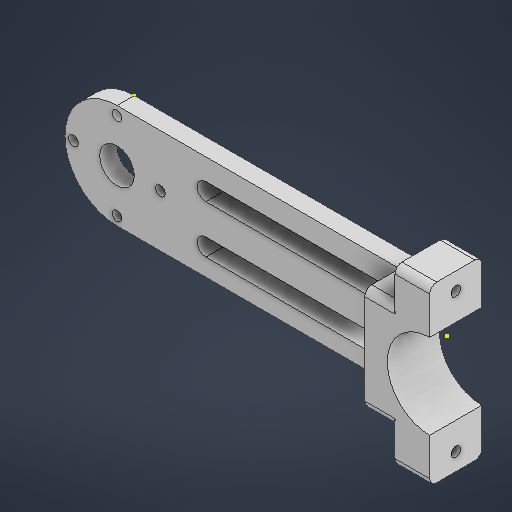
# Autodesk Inventor part: link1
Saved by Autodesk Inventor 2026.1 (Build 301233020, 233B)
## iProperties
Created: 2026-04-16
Part Number: link1
Material: Generic
Document SubType Name: Modeling
Designer: kadir
Density: 1 g/cm^3
Appearance: Default
Author: kadir
Autodesk Inventor part; units mm, degrees
ref_plane "YZ Plane" through (0, 0, 0) normal (1, 0, 0) x (0, 1, 0)
ref_plane "XZ Plane" through (0, 0, 0) normal (0, 1, 0) x (-1, 0, 0)
ref_plane "XY Plane" through (0, 0, 0) normal (0, 0, 1) x (1, 0, 0)
sketch "Sketch1" plane through (0, 0, 0) normal (0, 0, 1) x (1, 0, 0)
  circle A0 centre (0, 0) radius 15
  circle A1 centre (0, 0) radius 5
  circle A2 centre (-12.5, 0) radius 1.4
  circle A3 centre (0, -12.5) radius 1.4
  circle A4 centre (12.5, 0) radius 1.4
  circle A5 centre (0, 12.5) radius 1.4
  line L0 (0, -15) -> (1.0439, -14.9636)
  line L1 (100, 15) -> (70, 15)
  line L2 (70, -12.5614) -> (70, -15)
  line L3 (70, -15) -> (100, -15)
  line L4 (100, -15) -> (100, 15)
  line L5 (100, 15) -> (70, -15) construction
  line L6 (70, 15) -> (100, -15) construction
  circle A6 centre (100, 0) radius 12.2
  line L7 (0, 15) -> (100, 15)
  line L8 (0, -15) -> (100, -15)
  point P0 (85, 0)
  point P1 (100, -12.2)
  point P2 (100, 12.2)
  dimension "d0" = 30
  dimension "d1" = 10
  dimension "d2" = 2.8
  dimension "d3" = 12.5
  dimension "d6" = 360
  dimension "d9" = 30
  dimension "d10" = 30
  dimension "d11" = 24.4
  dimension "d12" = 100
  constraints: 18 end point, 7 centre point, 3 midpoint, 3 point on circle, 2 coincident, 2 horizontal alignment, 2 parallel, 1 horizontal, 1 perpendicular, 1 point on line, 1 tangent, 9 other
  measures "d0" diameter of A0
  measures "d1" diameter of A1
  measures "d2" diameter of A2
  measures "d3" distance of point (0, 0) A2.centre
  measures "d9" distance of L3.end L2.end
  measures "d10" distance of L2.end L1.end
  measures "d11" diameter of A6
  measures "d12" distance of A6.centre point (0, 0)
extrude "Extrusion1" add sketch "Sketch1" along normal blind 5 contours A0 L0 | A0 L7 L1 L4 A6 L3 L8 picked at (9.3778, -4.158)
sketch "Sketch2" plane through (0, 15, 0) normal (0, 1, 0) x (1, 0, 0)
  point P0 (0, 0)
sketch "Sketch3" plane through (0, 0, 5) normal (0, 0, 1) x (1, 0, 0)
  line L0 (100, 15) -> (0, 15) projected
  line L1 (0, -15) -> (100, -15) projected
  line L2 (81.3075, 15) -> (100, 15)
  line L3 (100, 15) -> (100, -15)
  line L4 (100, -15) -> (81.3075, -15)
  line L5 (81.3075, -15) -> (81.3075, 15)
  circle A0 centre (100, 0) radius 12.2
  point P0 (0, 0)
  point P1 (100, -12.2)
  point P2 (100, 12.2)
  dimension "d15" = 24.4
  constraints: 8 end point, 2 parallel, 1 centre point, 1 horizontal, 1 midpoint, 1 perpendicular, 1 point on line
  measures "d15" diameter of A0
extrude "Extrusion2" add sketch "Sketch3" along normal blind 10 contours L3 A0 L1 L5 L0
sketch "Sketch4" plane through (0, 15, 0) normal (0, 1, 0) x (1, 0, 0)
  line L0 (100, 0) -> (100, -15) projected
  line L1 (100, 0) -> (87.8, 0) projected
  line L2 (100, -15) -> (90, -15)
  line L3 (90, -15) -> (90, 0)
  line L4 (90, 0) -> (100, 0)
  line L5 (100, 0) -> (100, -15)
  point P0 (0, 0)
  dimension "d18" = 10
  constraints: 8 end point, 2 parallel, 1 horizontal, 1 perpendicular, 1 point on line
  measures "d18" distance of L3.end L4.end
extrude "Extrusion3" add sketch "Sketch4" along normal blind 10
sketch "Sketch5" plane through (0, -15, 0) normal (0, -1, 0) x (1, 0, 0)
  line L0 (100, 0) -> (100, 15) projected
  line L1 (100, 15) -> (90, 15)
  line L2 (90, 15) -> (90, 0)
  line L3 (90, 0) -> (100, 0)
  line L4 (100, 0) -> (100, 15)
  point P0 (0, 0)
  dimension "d21" = 10
  dimension "d22" = 15
  constraints: 8 end point, 2 parallel, 1 horizontal, 1 perpendicular
  measures "d21" distance of L3.end L2.end
  measures "d22" distance of L2.end L1.end
extrude "Extrusion4" add sketch "Sketch5" along normal blind 10
sketch "Sketch6" plane through (100, -12.2, 15) normal (1, 0, 0) x (0, 0, -1)
  circle A0 centre (7.5, -7.8) radius 1.4
  line L0 (15, -12.8) -> (0, -12.8) projected
  line L1 (0, 0) -> (0, -12.8) projected
  line L2 (15, 12.2) -> (0, 12.2)
  line L3 (0, 0) -> (0, 24.4) projected
  circle A1 centre (7.5, 32.2) radius 1.4
  dimension "d25" = 2.8
  dimension "d26" = 5
  dimension "d27" = 7.5
  constraints: 2 centre point, 2 end point, 1 midpoint, 1 symmetric about line, 1 other
  measures "d25" diameter of A0
  measures "d26" distance from line of L0 A0.centre
  measures "d27" distance from line of L1 A0.centre
extrude "Extrusion5" cut sketch "Sketch6" against normal through all
fillet "Fillet1" radius 2 2 edges at (95, -25, 0) (95, -25, 15)
fillet "Fillet2" radius 2 2 edges at (95, 25, 0) (95, 25, 15)
sketch "Sketch7" plane through (0, 0, 0) normal (0, 0, -1) x (-1, 0, 0)
  line L0 (-81.3075, 15) -> (-81.3075, -15) projected
  line L1 (-17.3755, -15) -> (-81.3075, -15)
  line L2 (-81.3075, -15) -> (-81.3075, 15)
  line L3 (-81.3075, 15) -> (-17.3755, 15)
  line L4 (-17.3755, 15) -> (-17.3755, -15)
  line L5 (-25.565, -7.4736) -> (-75.565, -7.4736) construction
  line L6 (-25.565, -4.9736) -> (-75.565, -4.9736)
  line L7 (-75.565, -9.9736) -> (-25.565, -9.9736)
  arc A0 (-25.565, -9.9736) -> (-25.565, -4.9736) centre (-25.565, -7.4736) ccw
  arc A1 (-75.565, -4.9736) -> (-75.565, -9.9736) centre (-75.565, -7.4736) ccw
  line L8 (-25.565, 6.3477) -> (-75.565, 6.3477) construction
  line L9 (-25.565, 3.8477) -> (-75.565, 3.8477)
  line L10 (-75.565, 8.8477) -> (-25.565, 8.8477)
  arc A2 (-25.565, 3.8477) -> (-25.565, 8.8477) centre (-25.565, 6.3477) ccw
  arc A3 (-75.565, 8.8477) -> (-75.565, 3.8477) centre (-75.565, 6.3477) ccw
  point P0 (0, 0)
  point P1 (-50.565, -7.4736)
  point P2 (-50.565, 6.3477)
  dimension "d32" = 30
  dimension "d33" = 5
  dimension "d34" = 50
  dimension "d35" = 50
  dimension "d36" = 2.5
  constraints: 24 end point, 8 point on circle, 8 tangent, 4 centre point, 4 parallel, 3 horizontal, 2 midpoint, 1 perpendicular, 1 vertical alignment
  measures "d32" distance of L3.end L1.start
  measures "d33" diameter of A1
  measures "d34" distance of L7.start L7.end
  measures "d35" distance of L10.start L10.end
  measures "d36" radius of A2
extrude "Extrusion6" cut sketch "Sketch7" against normal through all contours A0 L7 A1 L6 | L9 A3 L10 A2
fillet "Fillet3" radius 2 2 edges at (85.6537, 15, 15) (85.6537, -15, 15)
sketch "Sketch8" plane through (90, 15, 0) normal (-1, 0, 0) x (0, 0, 1)
  point P0 (0, -15)
body "Solid1"
